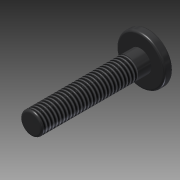
# Autodesk Inventor part: M5x25 low profile screw
Saved by Autodesk Inventor 2014 SP1 (Build 180222100, 222)
## iProperties
Created: 2016-04-10
Part Number: M5x25 low profile screw
Material: Generic
Document SubType Name: Modeling
Designer: Ben
Density: 1 g/cm^3
Appearance: Default
Author: Ben
Autodesk Inventor part; units mm, degrees
ref_plane "YZ Plane" through (0, 0, 0) normal (1, 0, 0) x (0, 1, 0)
ref_plane "XZ Plane" through (0, 0, 0) normal (0, 1, 0) x (-1, 0, 0)
ref_plane "XY Plane" through (0, 0, 0) normal (0, 0, 1) x (1, 0, 0)
sketch "Sketch1" plane through (0, 0, 0) normal (1, 0, 0) x (0, 1, 0)
  line L0 (0, 0) -> (5.5, 0)
  line L1 (5.5, 0) -> (5.5, 2)
  line L2 (5.5, 2) -> (2.5, 2)
  line L3 (2.5, 2) -> (2.5, 27)
  line L4 (2.5, 27) -> (0, 27)
  line L5 (0, 27) -> (0, 0)
  dimension "d0" = 25
  dimension "d1" = 2
  dimension "d2" = 5.5
  dimension "d3" = 2.5
  constraints: 12 end point, 4 parallel, 1 horizontal, 1 perpendicular
  measures "d0" distance between parallel lines of L2 L4
  measures "d1" distance of L0.end L1.end
  measures "d2" distance between parallel lines of L5 L1
  measures "d3" distance of L3.end L4.end
revolve "Revolution1" add sketch "Sketch1" angle 360 about axis through (0, 0, 27) along (0, 0, -1)
fillet "Fillet1" radius 0.5 3 edges at (0, -5.5, 0) (0, -5.5, 2) (0, -2.5, 27)
sketch "Sketch2" plane through (0, 0, 0) normal (0, 0, -1) x (-1, 0, 0)
  circle A0 centre (0, 0) radius 5 projected
  line L0 (1.5, -0.866) -> (0, -1.7321)
  line L1 (0, -1.7321) -> (-1.5, -0.866)
  line L2 (-1.5, -0.866) -> (-1.5, 0.866)
  line L3 (-1.5, 0.866) -> (0, 1.7321)
  line L4 (0, 1.7321) -> (1.5, 0.866)
  line L5 (1.5, 0.866) -> (1.5, -0.866)
  dimension "d6" = 3
  constraints: 12 end point, 1 coincident, 13 other
  measures "d6" distance between parallel lines of L5 L2
extrude "Extrusion1" cut sketch "Sketch2" against normal blind 3 contours L0 L1 L2 L3 L4 L5
thread "Thread1" size "M5x0.8" class "6g" standard "ANSI Metric M Profile" length 30 offset 3
body "Solid1"
